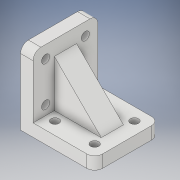
# Autodesk Inventor part: GearboxBrace
Saved by Autodesk Inventor 2019.4 (Build 234330000, 330)
## iProperties
Created: 2020-02-08
Part Number: GearboxBrace
Material: ABS Plastic
Document SubType Name: Modeling
Designer: Paul Lefeuvre
Density: 1.06 g/cm^3
Appearance: Smooth - White
Author: Paul Lefeuvre
Autodesk Inventor part; units mm, degrees
ref_plane "YZ Plane" through (0, 0, 0) normal (1, 0, 0) x (0, 1, 0)
ref_plane "XZ Plane" through (0, 0, 0) normal (0, 1, 0) x (-1, 0, 0)
sketch "Sketch1" plane through (0, 0, 0) normal (1, 0, 0) x (0, 1, 0)
  line L0 (-23.7, 20.7) -> (18.7, 20.7)
  line L1 (23.7, 15.7) -> (23.7, -15.7)
  line L2 (18.7, -20.7) -> (-23.7, -20.7)
  line L3 (-23.7, -20.7) -> (-23.7, 20.7)
  line L4 (-23.7, 20.7) -> (23.7, -20.7) construction
  line L5 (23.7, 20.7) -> (-23.7, -20.7) construction
  circle A0 centre (15.7, 12.7) radius 2.6
  circle A1 centre (15.7, -12.7) radius 2.6
  circle A2 centre (-9.7, 12.7) radius 2.6
  circle A3 centre (-9.7, -12.7) radius 2.6
  arc A4 (23.7, 15.7) -> (18.7, 20.7) centre (18.7, 15.7) ccw
  arc A5 (18.7, -20.7) -> (23.7, -15.7) centre (18.7, -15.7) ccw
  line L6 (-15.7, 20.7) -> (-15.7, -20.7)
  point P0 (0, 0)
  dimension "d0" = 5.2
  dimension "d1" = 5.2
  dimension "d2" = 5.2
  dimension "d3" = 5.2
  dimension "d5" = 25.4
  dimension "d6" = 25.4
  dimension "d7" = 25.4
  dimension "d8" = 25.4
  dimension "d9" = 14
  dimension "d10" = 8
  dimension "d11" = 8
  dimension "d13" = 8
  dimension "d14" = 8
  dimension "d15" = 8
  dimension "d16" = 5
  dimension "d17" = 8
  constraints: 14 end point, 6 centre point, 6 point on line, 4 point on circle, 4 tangent, 2 midpoint, 2 parallel, 2 perpendicular, 1 equal radius, 1 horizontal
  measures "d0" diameter of A0
  measures "d1" diameter of A1
  measures "d2" diameter of A2
  measures "d3" diameter of A3
  measures "d5" distance of A1.centre A0.centre
  measures "d6" distance of A2.centre A0.centre
  measures "d7" distance of A2.centre A3.centre
  measures "d8" distance of A1.centre A3.centre
  measures "d9" distance from line of L3 A3.centre
  measures "d10" distance from line of L2 A3.centre
  measures "d11" distance from line of L2 A1.centre
  measures "d13" distance from line of L1 A1.centre
  measures "d14" distance from line of L1 A0.centre
  measures "d15" distance from line of L0 A0.centre
  measures "d16" radius of A4
  measures "d17" distance between parallel lines of L3 L6
extrude "Extrusion1" add sketch "Sketch1" along normal blind 8
extrude "Extrusion2" add sketch "Sketch1" along normal blind 47.4 contours L0 L6 L2 L3
sketch "Sketch2" plane through (0, -23.7, -20.7) normal (0, -1, 0) x (1, 0, 0)
  circle A0 centre (39.4, 33.4) radius 2.6
  circle A1 centre (39.4, 8) radius 2.6
  circle A2 centre (14, 33.4) radius 2.6
  circle A3 centre (14, 8) radius 2.6
  line L0 (47.4, 41.4) -> (47.4, 0) projected
  line L1 (0, 41.4) -> (47.4, 41.4) projected
  line L2 (0, 0) -> (47.4, 0) projected
  line L3 (0, 41.4) -> (0, 0) projected
  line L4 (47.4, 0) -> (47.4, 41.4) projected
  arc A4 (47.4, 36.4) -> (42.4, 41.4) centre (42.4, 36.4) ccw
  arc A5 (42.4, 0) -> (47.4, 5) centre (42.4, 5) ccw
  line L5 (8, 41.4) -> (47.4, 41.4) projected
  line L6 (42.4, 41.4) -> (47.4, 41.4)
  line L7 (47.4, 41.4) -> (47.4, 36.4)
  line L8 (47.4, 5) -> (47.4, 0)
  line L9 (8, 0) -> (47.4, 0) projected
  line L10 (42.4, 0) -> (47.4, 0)
  point P0 (0, 20.7)
  dimension "d22" = 5.2
  dimension "d23" = 5.2
  dimension "d24" = 5.2
  dimension "d25" = 5.2
  dimension "d26" = 8
  dimension "d27" = 8
  dimension "d28" = 8
  dimension "d29" = 8
  dimension "d30" = 8
  dimension "d31" = 8
  dimension "d32" = 14
  dimension "d33" = 14
  dimension "d34" = 5
  dimension "d35" = 5
  constraints: 8 end point, 6 centre point, 4 point on circle, 4 point on line, 4 tangent, 1 collinear, 1 horizontal, 1 perpendicular
  measures "d22" diameter of A0
  measures "d23" diameter of A1
  measures "d24" diameter of A3
  measures "d25" diameter of A2
  measures "d26" distance from line of L0 A0.centre
  measures "d27" distance from line of L1 A0.centre
  measures "d28" distance from line of L0 A1.centre
  measures "d29" distance from line of L2 A1.centre
  measures "d30" distance from line of L1 A2.centre
  measures "d31" distance from line of L2 A3.centre
  measures "d32" distance from line of L3 A2.centre
  measures "d33" distance from line of L3 A3.centre
  measures "d34" radius of A4
  measures "d35" radius of A5
extrude "Extrusion3" cut sketch "Sketch2" against normal blind 10 contours A0 | A1 | A2 | A3 | L0 A4 L1 | L0 L2 A5
ref_plane "Work Plane4" through (8, 18.7, -7.1) normal (0, 0, -1) x (-1, 0, 0)
sketch "Sketch6" plane through (8, 18.7, -7.1) normal (0, 0, -1) x (-1, 0, 0)
  line L0 (0, -34.4) -> (-34.4, -34.4) projected
  line L1 (-30, -34.4) -> (0, -4.4)
  line L2 (0, -34.4) -> (0, 0) projected
  line L3 (-30, -34.4) -> (12.4264, -34.4) construction
  point P0 (8, -18.7)
  dimension "d50" = 45
  dimension "d51" = 30
  constraints: 4 end point, 2 point on line, 1 equal length, 1 horizontal
  measures "d50" angle of L3 L1
  measures "d51" horizontal distance of L1.start L1.end
extrude "Extrusion7" add sketch "Sketch6" against normal blind 14.2
equation "\"d27\" = d26"
equation "\"d28\" = d26"
equation "\"d29\" = d26"
equation "\"d30\" = d26"
equation "\"d31\" = d26"
equation "\"d33\" = d32"
body "Solid1"
